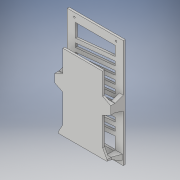
# Autodesk Inventor part: Robotics Club
Saved by Autodesk Inventor 2018 (Build 220112000, 112)
## iProperties
Created: 2018-10-30
Part Number: Robotics Club
Material: Generic
Document SubType Name: Modeling
Designer: 109307
Density: 1 g/cm^3
Appearance: Default
Author: 109307
Autodesk Inventor part; units mm, degrees
ref_plane "YZ Plane" through (0, 0, 0) normal (1, 0, 0) x (0, 1, 0)
sketch "Sketch1" plane through (0, 0, 0) normal (0, 0, 1) x (1, 0, 0)
  line L0 (0, 0) -> (-169.8625, 0)
  line L1 (-169.8625, 0) -> (-169.8625, 87.884)
  line L2 (-169.8625, 87.884) -> (0, 87.884)
  line L3 (0, 87.884) -> (0, 0)
  circle A0 centre (-163.5125, 11.176) radius 1.27
  circle A1 centre (-163.5125, 76.708) radius 1.27
  circle A2 centre (-6.35, 76.708) radius 1.27
  circle A3 centre (-6.35, 11.176) radius 1.27
  dimension "d0" = 169.8625
  dimension "d1" = 87.884
  dimension "d2" = 2.54
  dimension "d3" = 2.54
  dimension "d4" = 2.54
  dimension "d5" = 2.54
  dimension "d6" = 11.176
  dimension "d7" = 6.35
  dimension "d8" = 6.35
  dimension "d9" = 11.176
  dimension "d10" = 11.176
  dimension "d11" = 11.176
  dimension "d12" = 6.35
  dimension "d13" = 6.35
  constraints: 8 end point, 4 centre point, 2 parallel, 1 horizontal, 1 perpendicular
  measures "d0" distance of L1.end L2.end
  measures "d1" distance of L0.end L1.end
  measures "d2" diameter of A0
  measures "d3" diameter of A1
  measures "d4" diameter of A2
  measures "d5" diameter of A3
  measures "d6" distance from line of L2 A1.centre
  measures "d7" distance from line of L1 A1.centre
  measures "d8" distance from line of L1 A0.centre
  measures "d9" distance from line of L0 A0.centre
  measures "d10" distance from line of L0 A3.centre
  measures "d11" distance from line of L2 A2.centre
  measures "d12" distance from line of L3 A2.centre
  measures "d13" distance from line of L3 A3.centre
extrude "Extrusion1" add sketch "Sketch1" along normal blind 3.175
sketch "Sketch2" plane through (0, 0, 3.175) normal (0, 0, 1) x (1, 0, 0)
  line L0 (-24.6112, 71.9836) -> (-109.5742, 71.9836) construction
  line L1 (-109.5742, 71.9836) -> (-109.5742, 15.9004) construction
  line L2 (-109.5742, 15.9004) -> (-24.6112, 15.9004) construction
  line L3 (-24.6112, 15.9004) -> (-24.6112, 71.9836) construction
  circle A0 centre (-86.0284, 68.5292) radius 1.3335
  circle A1 centre (-86.0284, 19.3548) radius 1.3335
  circle A2 centre (-28.0656, 19.3548) radius 1.3335
  circle A3 centre (-28.0656, 68.5292) radius 1.3335
  line L4 (-169.8625, 0) -> (0, 0) projected
  line L5 (0, 87.884) -> (-169.8625, 87.884) projected
  dimension "d16" = 84.963
  dimension "d17" = 56.0832
  dimension "d18" = 2.667
  dimension "d19" = 2.667
  dimension "d20" = 2.667
  dimension "d21" = 2.667
  dimension "d22" = 23.5458
  dimension "d23" = 23.5458
  dimension "d24" = 3.4544
  dimension "d25" = 3.4544
  dimension "d26" = 3.4544
  dimension "d27" = 3.4544
  dimension "d28" = 3.4544
  dimension "d29" = 3.4544
  dimension "d30" = 15.9004
  dimension "d31" = 15.9004
  constraints: 8 end point, 4 centre point, 2 parallel, 1 horizontal, 1 perpendicular
  measures "d16" distance of L2.end L1.end
  measures "d17" distance of L1.end L0.end
  measures "d18" diameter of A0
  measures "d19" diameter of A1
  measures "d20" diameter of A2
  measures "d21" diameter of A3
  measures "d22" distance from line of L1 A1.centre
  measures "d23" distance from line of L1 A0.centre
  measures "d24" distance from line of L2 A1.centre
  measures "d25" distance from line of L0 A0.centre
  measures "d26" distance from line of L2 A2.centre
  measures "d27" distance from line of L0 A3.centre
  measures "d28" distance from line of L3 A3.centre
  measures "d29" distance from line of L3 A2.centre
  measures "d30" distance between parallel lines of L4 L2
  measures "d31" distance between parallel lines of L5 L0
sketch "Sketch4" plane through (0, 0, 3.175) normal (0, 0, 1) x (1, 0, 0)
  circle A0 centre (-6.35, 11.176) radius 1.27 projected
  circle A1 centre (-6.35, 76.708) radius 1.27 projected
  circle A2 centre (-163.5125, 76.708) radius 1.27 projected
  circle A3 centre (-163.5125, 11.176) radius 1.27 projected
  line L0 (-169.8625, 0) -> (0, 0) projected
  line L1 (0, 0) -> (0, 87.884) projected
  line L2 (0, 87.884) -> (-169.8625, 87.884) projected
  line L3 (-169.8625, 87.884) -> (-169.8625, 0) projected
  line L4 (-157.1625, 12.7) -> (-12.7, 12.7)
  line L5 (-12.7, 12.7) -> (-12.7, 75.184)
  line L6 (-12.7, 75.184) -> (-157.1625, 75.184)
  line L7 (-157.1625, 75.184) -> (-157.1625, 12.7)
  line L8 (-142.0749, 12.7) -> (-27.7749, 12.7) construction
  line L9 (-27.7749, 12.7) -> (-27.7749, 75.184)
  line L10 (-142.0749, 12.7) -> (-142.0749, 75.184)
  line L11 (-27.7749, 12.7) -> (-34.1249, 12.7) construction
  line L12 (-34.1249, 12.7) -> (-40.4749, 12.7) construction
  line L13 (-40.4749, 12.7) -> (-46.8249, 12.7) construction
  line L14 (-46.8249, 12.7) -> (-53.1749, 12.7) construction
  line L15 (-53.1749, 12.7) -> (-59.5249, 12.7) construction
  line L16 (-59.5249, 12.7) -> (-65.8749, 12.7) construction
  line L17 (-65.8749, 12.7) -> (-72.2249, 12.7) construction
  line L18 (-72.2249, 12.7) -> (-78.5749, 12.7) construction
  line L19 (-78.5749, 12.7) -> (-84.9249, 12.7) construction
  line L20 (-84.9249, 12.7) -> (-91.2749, 12.7) construction
  line L21 (-91.2749, 12.7) -> (-97.6249, 12.7) construction
  line L22 (-97.6249, 12.7) -> (-148.4249, 12.7) construction
  line L23 (-148.4249, 12.7) -> (-97.6249, 12.7) construction
  line L24 (-97.6249, 12.7) -> (-103.9749, 12.7) construction
  line L25 (-103.9749, 12.7) -> (-110.3249, 12.7) construction
  line L26 (-110.3249, 12.7) -> (-116.6749, 12.7) construction
  line L27 (-116.6749, 12.7) -> (-123.0249, 12.7) construction
  line L28 (-123.0249, 12.7) -> (-129.3749, 12.7) construction
  line L29 (-129.3749, 12.7) -> (-135.7249, 12.7) construction
  line L30 (-135.7249, 12.7) -> (-142.0749, 12.7) construction
  line L31 (-142.0749, 12.7) -> (-148.4249, 12.7) construction
  line L32 (-148.4249, 12.7) -> (-154.7749, 12.7) construction
  line L33 (-103.9749, 43.942) -> (-81.7499, 43.942) construction
  line L34 (-142.0749, 75.184) -> (-27.7749, 75.184) construction
  line L35 (-27.7749, 75.184) -> (-34.1249, 75.184) construction
  line L36 (-34.1249, 75.184) -> (-40.4749, 75.184) construction
  line L37 (-40.4749, 75.184) -> (-46.8249, 75.184) construction
  line L38 (-46.8249, 75.184) -> (-53.1749, 75.184) construction
  line L39 (-53.1749, 75.184) -> (-59.5249, 75.184) construction
  line L40 (-59.5249, 75.184) -> (-65.8749, 75.184) construction
  line L41 (-65.8749, 75.184) -> (-72.2249, 75.184) construction
  line L42 (-72.2249, 75.184) -> (-78.5749, 75.184) construction
  line L43 (-78.5749, 75.184) -> (-84.9249, 75.184) construction
  line L44 (-84.9249, 75.184) -> (-91.2749, 75.184) construction
  line L45 (-91.2749, 75.184) -> (-97.6249, 75.184) construction
  line L46 (-97.6249, 75.184) -> (-103.9749, 75.184) construction
  line L47 (-103.9749, 75.184) -> (-110.3249, 75.184) construction
  line L48 (-110.3249, 75.184) -> (-116.6749, 75.184) construction
  line L49 (-116.6749, 75.184) -> (-123.0249, 75.184) construction
  line L50 (-123.0249, 75.184) -> (-129.3749, 75.184) construction
  line L51 (-129.3749, 75.184) -> (-135.7249, 75.184) construction
  line L52 (-135.7249, 75.184) -> (-142.0749, 75.184) construction
  line L53 (-34.1249, 12.7) -> (-40.4749, 75.184)
  line L54 (-27.7749, 12.7) -> (-34.1249, 75.184)
  line L55 (-40.4749, 12.7) -> (-46.8249, 75.184)
  line L56 (-46.8249, 12.7) -> (-53.1749, 75.184)
  line L57 (-53.1749, 12.7) -> (-59.5249, 75.184)
  line L58 (-59.5249, 12.7) -> (-65.8749, 75.184)
  line L59 (-65.8749, 12.7) -> (-72.2249, 75.184)
  line L60 (-72.2249, 12.7) -> (-78.5749, 75.184)
  line L61 (-78.5749, 12.7) -> (-84.9249, 75.184)
  line L62 (-84.9249, 12.7) -> (-91.2749, 75.184)
  line L63 (-91.2749, 12.7) -> (-97.6249, 75.184)
  line L64 (-97.6249, 12.7) -> (-103.9749, 75.184)
  line L65 (-103.9749, 12.7) -> (-110.3249, 75.184)
  line L66 (-110.3249, 12.7) -> (-116.6749, 75.184)
  line L67 (-116.6749, 12.7) -> (-123.0249, 75.184)
  line L68 (-123.0249, 12.7) -> (-129.3749, 75.184)
  line L69 (-129.3749, 12.7) -> (-135.7249, 75.184)
  line L70 (-135.7249, 12.7) -> (-142.0749, 75.184)
  line L71 (-27.7749, 12.7) -> (-34.1249, 12.7)
  line L72 (-40.4749, 12.7) -> (-34.1249, 12.7)
  line L73 (-46.8249, 12.7) -> (-40.4749, 12.7)
  line L74 (-53.1749, 12.7) -> (-46.8249, 12.7)
  line L75 (-59.5249, 12.7) -> (-53.1749, 12.7)
  line L76 (-65.8749, 12.7) -> (-59.5249, 12.7)
  line L77 (-72.2249, 12.7) -> (-65.8749, 12.7)
  line L78 (-142.0749, 12.7) -> (-72.2249, 12.7)
  line L79 (-78.5749, 12.7) -> (-84.9249, 12.7)
  line L80 (-84.9249, 12.7) -> (-91.2749, 12.7)
  line L81 (-91.2749, 12.7) -> (-97.6249, 12.7)
  line L82 (-97.6249, 12.7) -> (-103.9749, 12.7)
  line L83 (-110.3249, 12.7) -> (-103.9749, 12.7)
  line L84 (-116.6749, 12.7) -> (-110.3249, 12.7)
  line L85 (-123.0249, 12.7) -> (-116.6749, 12.7)
  line L86 (-129.3749, 12.7) -> (-123.0249, 12.7)
  line L87 (-129.3749, 12.7) -> (-135.7249, 12.7)
  line L88 (-135.7249, 12.7) -> (-142.0749, 12.7)
  line L89 (-27.7749, 75.184) -> (-34.1249, 75.184)
  line L90 (-34.1249, 75.184) -> (-40.4749, 75.184)
  line L91 (-40.4749, 75.184) -> (-46.8249, 75.184)
  line L92 (-46.8249, 75.184) -> (-53.1749, 75.184)
  line L93 (-53.1749, 75.184) -> (-59.5249, 75.184)
  line L94 (-59.5249, 75.184) -> (-65.8749, 75.184)
  line L95 (-72.2249, 75.184) -> (-65.8749, 75.184)
  line L96 (-72.2249, 75.184) -> (-78.5749, 75.184)
  line L97 (-78.5749, 75.184) -> (-84.9249, 75.184)
  line L98 (-84.9249, 75.184) -> (-91.2749, 75.184)
  line L99 (-91.2749, 75.184) -> (-97.6249, 75.184)
  line L100 (-97.6249, 75.184) -> (-103.9749, 75.184)
  line L101 (-103.9749, 75.184) -> (-110.3249, 75.184)
  line L102 (-110.3249, 75.184) -> (-116.6749, 75.184)
  line L103 (-116.6749, 75.184) -> (-123.0249, 75.184)
  line L104 (-129.3749, 75.184) -> (-123.0249, 75.184)
  line L105 (-129.3749, 75.184) -> (-135.7249, 75.184)
  line L106 (-135.7249, 75.184) -> (-142.0749, 75.184)
  line L107 (-142.0749, 12.7) -> (-135.7249, 12.7)
  line L108 (-135.7249, 12.7) -> (-142.0749, 12.7)
  line L109 (-142.0749, 12.7) -> (-142.0749, 75.184)
  line L110 (-142.0749, 75.184) -> (-135.7249, 12.7)
  line L111 (-84.9249, 12.7) -> (-91.2749, 12.7)
  line L112 (-91.2749, 12.7) -> (-97.6249, 75.184)
  line L113 (-97.6249, 75.184) -> (-91.2749, 75.184)
  line L114 (-91.2749, 75.184) -> (-84.9249, 12.7)
  dimension "d48" = 12.7
  dimension "d49" = 114.3
  dimension "d50" = 15.0876
  dimension "d51" = 6.35
  dimension "d52" = 6.35
  dimension "d53" = 6.35
  dimension "d54" = 6.35
  dimension "d55" = 6.35
  dimension "d56" = 6.35
  dimension "d57" = 6.35
  dimension "d58" = 6.35
  dimension "d59" = 6.35
  dimension "d60" = 6.35
  dimension "d61" = 6.35
  dimension "d64" = 6.35
  dimension "d65" = 6.35
  dimension "d66" = 6.35
  dimension "d67" = 6.35
  dimension "d68" = 6.35
  dimension "d69" = 6.35
  dimension "d70" = 6.35
  constraints: 216 end point, 35 collinear, 19 symmetric about line, 6 horizontal, 6 point on line, 3 perpendicular, 42 other
  measures "d48" distance between parallel lines of L3 L7
  measures "d49" distance of L10.start L9.start
  measures "d50" distance from line of L7 L10.start
  measures "d51" distance of L9.start L11.end
  measures "d52" distance of L11.end L12.end
  measures "d53" distance of L12.end L13.end
  measures "d54" distance of L13.end L14.end
  measures "d55" distance of L14.end L15.end
  measures "d56" distance of L15.end L16.end
  measures "d57" distance of L16.end L17.end
  measures "d58" distance of L17.end L18.end
  measures "d59" distance of L18.end L19.end
  measures "d60" distance of L19.end L20.end
  measures "d61" distance of L20.end L21.end
  measures "d64" distance of L21.end L24.end
  measures "d65" distance of L24.end L25.end
  measures "d66" distance of L25.end L26.end
  measures "d67" distance of L26.end L27.end
  measures "d68" distance of L27.end L28.end
  measures "d69" distance of L28.end L29.end
  measures "d70" distance of L29.end L30.end
sketch "Sketch5" plane through (0, 0, 3.175) normal (0, 0, 1) x (1, 0, 0)
  line L0 (-27.7749, 12.7) -> (-27.7749, 75.184) projected
  circle A0 centre (-6.35, 11.176) radius 1.27 projected
  circle A1 centre (-6.35, 76.708) radius 1.27 projected
  circle A2 centre (-163.5125, 76.708) radius 1.27 projected
  circle A3 centre (-163.5125, 11.176) radius 1.27 projected
  line L1 (-169.8625, 0) -> (0, 0) projected
  line L2 (0, 0) -> (0, 87.884) projected
  line L3 (0, 87.884) -> (-169.8625, 87.884) projected
  line L4 (-169.8625, 87.884) -> (-169.8625, 0) projected
  line L5 (-12.7, 12.7) -> (-12.7, 75.184) projected
  line L6 (-157.1625, 12.7) -> (-12.7, 12.7) projected
  line L7 (-34.1249, 12.7) -> (-40.4749, 75.184) projected
  line L8 (-27.7749, 12.7) -> (-34.1249, 75.184) projected
  line L9 (-40.4749, 12.7) -> (-46.8249, 75.184) projected
  line L10 (-46.8249, 12.7) -> (-53.1749, 75.184) projected
  line L11 (-53.1749, 12.7) -> (-59.5249, 75.184) projected
  line L12 (-59.5249, 12.7) -> (-65.8749, 75.184) projected
  line L13 (-65.8749, 12.7) -> (-72.2249, 75.184) projected
  line L14 (-72.2249, 12.7) -> (-78.5749, 75.184) projected
  line L15 (-78.5749, 12.7) -> (-84.9249, 75.184) projected
  line L16 (-84.9249, 12.7) -> (-91.2749, 75.184) projected
  line L17 (-91.2749, 12.7) -> (-97.6249, 75.184) projected
  line L18 (-97.6249, 12.7) -> (-103.9749, 75.184) projected
  line L19 (-103.9749, 12.7) -> (-110.3249, 75.184) projected
  line L20 (-103.9749, 43.942) -> (-81.7499, 43.942) construction
  line L21 (-142.0749, 12.7) -> (-142.0749, 75.184) projected
  line L22 (-157.1625, 75.184) -> (-157.1625, 12.7) projected
  line L23 (-12.7, 75.184) -> (-157.1625, 75.184) projected
  line L24 (-142.0749, 12.7) -> (-142.0749, 75.184) projected
  line L25 (-135.7249, 12.7) -> (-142.0749, 75.184) projected
  line L26 (-129.3749, 12.7) -> (-135.7249, 75.184) projected
  line L27 (-123.0249, 12.7) -> (-129.3749, 75.184) projected
  line L28 (-116.6749, 12.7) -> (-123.0249, 75.184) projected
  line L29 (-110.3249, 12.7) -> (-116.6749, 75.184) projected
  line L30 (-142.0749, 75.184) -> (-27.7749, 75.184) construction
  line L31 (-142.0749, 12.7) -> (-27.7749, 12.7) construction
  constraints: 4 other
extrude "Extrusion2" cut sketch "Sketch5" against normal blind 3.175 contours L8 L23 L0 | L0 L23 L5 L6 | L6 L9 L23 L7 | L6 L11 L23 L10 | L6 L13 L23 L12 | L6 L15 L23 L14 | L6 L17 L23 L16 | L6 L19 L23 L18 | L6 L28 L23 L29 | L6 L26 L23 L27 | L6 L25 L23 L26 | L6 L21 L25 | L6 L22 L23 L21
sketch "Sketch6" plane through (0, 0, 3.175) normal (0, 0, 1) x (1, 0, 0)
  line L0 (-157.1625, 75.184) -> (-129.3749, 75.184) projected
  line L1 (-129.3749, 75.184) -> (-135.7249, 75.184)
  line L2 (-157.1625, 12.7) -> (-123.0249, 12.7) projected
  line L3 (-123.0249, 12.7) -> (-129.3749, 12.7)
  line L4 (-129.3749, 12.7) -> (-135.7249, 12.7)
  line L5 (-135.7249, 75.184) -> (-142.0749, 75.184)
  line L6 (-142.0749, 75.184) -> (-135.7249, 12.7)
  line L7 (-129.3749, 12.7) -> (-135.7249, 75.184)
  point P0 (0, 0)
  dimension "d75" = 6.35
  dimension "d76" = 6.35
  dimension "d77" = 6.35
  dimension "d78" = 6.35
  constraints: 12 end point, 4 point on line
  measures "d75" distance of L0.end L1.end
  measures "d76" distance of L2.end L3.end
  measures "d77" distance of L3.end L4.end
  measures "d78" distance of L1.end L5.end
extrude "Extrusion3" add sketch "Sketch6" against normal blind 3.175
sketch "Sketch7" plane through (0, 0, 3.175) normal (0, 0, 1) x (1, 0, 0)
  line L0 (-15.0876, 5.842) -> (-15.0876, 82.042) construction
  line L1 (-169.8625, 0) -> (0, 0) projected
  line L2 (-15.0876, 5.842) -> (-154.7876, 5.842) construction
  line L3 (-154.7876, 5.842) -> (-154.7876, 82.042) construction
  line L4 (-154.7876, 82.042) -> (-15.0876, 82.042) construction
  line L5 (-27.7749, 12.7) -> (-12.7, 12.7) projected
  line L6 (-15.0876, 5.842) -> (-12.7, 5.842)
  line L7 (-12.7, 5.842) -> (-12.7, 12.7)
  line L8 (-12.7, 12.7) -> (-15.0876, 12.7)
  line L9 (-15.0876, 12.7) -> (-15.0876, 5.842)
  line L10 (-12.7, 12.7) -> (-12.7, 75.184) projected
  line L11 (-15.0876, 82.042) -> (-12.7, 82.042)
  line L12 (-12.7, 82.042) -> (-12.7, 75.184)
  line L13 (-12.7, 75.184) -> (-15.0876, 75.184)
  line L14 (-15.0876, 75.184) -> (-15.0876, 82.042)
  line L15 (-84.9376, -43.7572) -> (-84.9376, 110.8857) construction
  line L16 (0, 0) -> (-169.8625, 0) projected
  line L17 (-84.9376, 5.842) -> (-91.2876, 5.842)
  line L18 (-91.2876, 5.842) -> (-91.2876, 0)
  line L19 (-91.2876, 0) -> (-84.9376, 0)
  line L20 (-84.9376, 0) -> (-78.5876, 0)
  line L21 (-78.5876, 0) -> (-78.5876, 5.842)
  line L22 (-78.5876, 5.842) -> (-84.9376, 5.842)
  line L23 (-84.9376, 82.042) -> (-91.2876, 82.042)
  line L24 (-91.2876, 82.042) -> (-91.2876, 87.884)
  line L25 (-169.8625, 87.884) -> (0, 87.884) projected
  line L26 (-91.2876, 87.884) -> (-78.5876, 87.884)
  line L27 (-78.5876, 87.884) -> (-78.5876, 82.042)
  line L28 (-84.9376, 82.042) -> (-78.5876, 82.042)
  dimension "d81" = 76.2
  dimension "d82" = 5.842
  dimension "d83" = 139.7
  dimension "d84" = 15.0876
  dimension "d85" = 0
  dimension "d86" = 0
  dimension "d89" = 6.35
  dimension "d90" = 12.7
  constraints: 48 end point, 8 perpendicular, 8 point on line, 6 parallel, 5 horizontal, 3 vertical, 2 midpoint
  measures "d81" distance of L0.start L0.end
  measures "d82" distance from line of L0.start L1
  measures "d83" distance of L2.start L2.end
  measures "d84" horizontal distance of L1.end L2.start
  measures "d85" distance from line of L2.start L0
  measures "d86" distance from line of L0.start L2
  measures "d89" distance of L23.start L23.end
  measures "d90" distance of L24.end L26.end
extrude "Extrusion4" add sketch "Sketch7" along normal blind 12.7 contours L5 L7 L6 L9 | L11 L12 L13 L14 | L23 L24 L25 L27 L28
ref_plane "Work Plane1" through (-169.8625, 43.942, 0) normal (0, 1, 0) x (1, 0, 0)
mirror "Mirror1" about plane through (-169.8625, 43.942, 0) normal (0, 1, 0) of "Extrusion4"
chamfer "Chamfer2" distance 12.7 angle 20 1 edges at (-13.8938, 5.842, 3.175) measured on face at (-13.8938, 5.842, 3.675)
chamfer "Chamfer3" distance 12.7 angle 20 1 edges at (-13.8938, 82.042, 3.175) measured on face at (-13.8938, 82.042, 3.675)
chamfer "Chamfer4" distance 12.7 angle 20 1 edges at (-78.5876, 84.963, 3.175) measured on face at (-78.5876, 84.963, 3.675)
chamfer "Chamfer5" distance 12.7 angle 20 1 edges at (-91.2876, 84.963, 3.175) measured on face at (-91.2876, 84.963, 3.675)
chamfer "Chamfer6" distance 12.7 angle 20 1 edges at (-91.2876, 2.921, 3.175) measured on face at (-91.2876, 2.921, 3.675)
chamfer "Chamfer7" distance 12.7 angle 20 1 edges at (-78.5876, 2.921, 3.175) measured on face at (-78.5876, 2.921, 3.675)
sketch "Sketch8" plane through (0, 0, 3.175) normal (0, 0, 1) x (1, 0, 0)
  circle A0 centre (-6.35, 11.176) radius 1.27 projected
  circle A1 centre (-6.35, 11.176) radius 3.175
  circle A2 centre (-6.35, 76.708) radius 1.27 projected
  circle A3 centre (-6.35, 76.708) radius 3.175
  point P0 (0, 0)
  dimension "d115" = 6.35
  dimension "d116" = 6.35
  constraints: 2 centre point, 2 coincident
  measures "d115" diameter of A1
  measures "d116" diameter of A3
extrude "Extrusion5" cut sketch "Sketch8" along normal blind 50.8
ref_plane "Work Plane2" through (0, 0, 19.685) normal (0, 0, 1) x (1, 0, 0)
sketch "Sketch10" plane through (0, 0, 19.685) normal (0, 0, 1) x (1, 0, 0)
  line L0 (-15.0876, 5.842) -> (-27.7749, 12.7) projected
  line L1 (-15.0876, 5.842) -> (-12.7, 5.842) projected
  line L2 (-12.7, 5.842) -> (-12.7, 12.7) projected
  line L3 (-12.7, 75.184) -> (-12.7, 12.7) projected
  line L4 (-12.7, 75.184) -> (-12.7, 82.042) projected
  line L5 (-12.7, 82.042) -> (-15.0876, 82.042) projected
  line L6 (-15.0876, 82.042) -> (-27.7749, 75.184) projected
  line L7 (-27.7749, 75.184) -> (-34.1249, 75.184) projected
  line L8 (-72.2249, 75.184) -> (-34.1249, 75.184) projected
  line L9 (-72.2249, 75.184) -> (-78.5876, 87.884) projected
  line L10 (-78.5876, 87.884) -> (-91.2876, 87.884) projected
  line L11 (-91.2876, 87.884) -> (-97.6249, 75.184) projected
  line L12 (-157.1625, 75.184) -> (-97.6249, 75.184) projected
  line L13 (-157.1625, 12.7) -> (-157.1625, 75.184) projected
  line L14 (-97.6249, 12.7) -> (-157.1625, 12.7) projected
  line L15 (-91.2876, 0) -> (-97.6249, 12.7) projected
  line L16 (-78.5876, 0) -> (-91.2876, 0) projected
  line L17 (-78.5876, 0) -> (-72.2249, 12.7) projected
  line L18 (-27.7749, 12.7) -> (-72.2249, 12.7) projected
  point P0 (0, 0)
extrude "Extrusion7" add sketch "Sketch10" along normal blind 3.175
sketch "Sketch11" plane through (0, 0, 15.875) normal (0, 0, 1) x (1, 0, 0)
  line L0 (-15.0876, 82.042) -> (-15.0876, 75.184) projected
  line L1 (-15.0876, 75.184) -> (-12.7, 75.184) projected
  line L2 (-12.7, 82.042) -> (-15.0876, 82.042) projected
  line L3 (-12.7, 12.7) -> (-15.0876, 12.7) projected
  line L4 (-15.0876, 12.7) -> (-15.0876, 5.842) projected
  line L5 (-15.0876, 5.842) -> (-12.7, 5.842) projected
  line L6 (-91.2876, 82.042) -> (-78.5876, 82.042) projected
  line L7 (-78.5876, 82.042) -> (-78.5876, 87.884) projected
  line L8 (-78.5876, 87.884) -> (-91.2876, 87.884) projected
  line L9 (-91.2876, 87.884) -> (-91.2876, 82.042) projected
  line L10 (-91.2876, 5.842) -> (-78.5876, 5.842) projected
  line L11 (-91.2876, 0) -> (-91.2876, 5.842) projected
  line L12 (-78.5876, 0) -> (-91.2876, 0) projected
  line L13 (-78.5876, 5.842) -> (-78.5876, 0) projected
  line L14 (-12.7, 5.842) -> (-12.7, 12.7) projected
  line L15 (-12.7, 75.184) -> (-12.7, 82.042) projected
  point P0 (0, 0)
extrude "Extrusion8" add sketch "Sketch11" along normal up to next
chamfer "Chamfer8" distance 3.175 angle 45 10 edges at (-15.0876, 9.271, 19.685) (-15.0876, 78.613, 19.685) (-13.8938, 75.184, 19.685) (-13.8938, 12.7, 19.685) (-84.9376, 5.842, 19.685) (-78.5876, 2.921, 19.685) (-84.9376, 82.042, 19.685) (-78.5876, 84.963, 19.685) (-91.2876, 2.921, 19.685) (-91.2876, 84.963, 19.685)
sketch "Sketch12" plane through (0, 0, 22.86) normal (0, 0, 1) x (1, 0, 0)
  line L0 (-157.1625, 75.184) -> (-131.7625, 75.184)
  line L1 (-157.1625, 75.184) -> (-97.6249, 75.184) projected
  line L2 (-131.7625, 75.184) -> (-131.7625, 12.7)
  line L3 (-97.6249, 12.7) -> (-157.1625, 12.7) projected
  line L4 (-157.1625, 12.7) -> (-157.1625, 75.184) projected
  line L5 (-157.1625, 12.7) -> (-131.7625, 12.7)
  line L6 (-157.1625, 75.184) -> (-157.1625, 12.7)
  point P0 (0, 0)
  dimension "d129" = 25.4
  constraints: 8 end point, 3 perpendicular, 2 point on line
  measures "d129" distance of L0.start L0.end
extrude "Extrusion9" cut sketch "Sketch12" against normal blind 3.175
chamfer "Chamfer9" distance 16.51 angle 20 1 edges at (-12.7, 6.9598, 3.175)
chamfer "Chamfer10" distance 16.51 angle 20 1 edges at (-12.7, 80.9242, 3.175)
sketch "Sketch13" plane through (0, 0, 3.175) normal (0, 0, 1) x (1, 0, 0)
  arc A0 (-6.6909, 9.9526) -> (-6.6909, 12.3994) centre (-6.35, 11.176) ccw projected
  arc A1 (-6.6909, 75.4846) -> (-6.6909, 77.9314) centre (-6.35, 76.708) ccw projected
  circle A2 centre (-6.35, 76.708) radius 3.175
  circle A3 centre (-6.35, 11.176) radius 3.175
  point P0 (0, 0)
  dimension "d138" = 6.35
  dimension "d139" = 6.35
  constraints: 2 centre point, 2 coincident
  measures "d138" diameter of A2
  measures "d139" diameter of A3
extrude "Extrusion10" cut sketch "Sketch13" along normal blind 50.8
body "Solid1"
